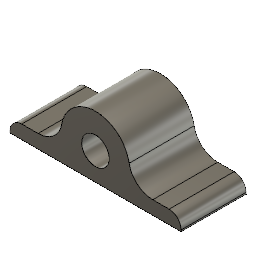
Rod Attach (Autodesk Fusion 360 design; units mm, degrees)
Autodesk Fusion 360 part; units mm, degrees
sketch "Sketch1" plane through (0, 0, 0) normal (0, 0, 1) x (1, 0, 0)
  circle A0 centre (0, 0) radius 4
  circle A1 centre (0, 0) radius 10
  line L0 (-25, -8) -> (25, -8)
  line L1 (25, -8) -> (25, -4)
  line L2 (25, -4) -> (-25, -4)
  line L3 (-25, -4) -> (-25, -8)
  line L4 (-25, -8) -> (25, -4) construction
  line L5 (25, -8) -> (-25, -4) construction
  circle A2 centre (-16.7332, 3) radius 7
  circle A3 centre (16.7332, 3) radius 7
  dimension "d1" = 8
  dimension "d2" = 20
  dimension "d3" = 50
  dimension "d4" = 4
  dimension "d5" = 14
  dimension "d6" = 14
  constraint coincident A0.centre A1.centre
  constraint perpendicular L0 L1
  constraint parallel L0 L2
  constraint parallel L1 L3
  constraint horizontal L0
  constraint tangent L2 A2
  constraint tangent A1 A2
  constraint tangent A1 A3
  constraint tangent L2 A3
  measures "d1" diameter of A0
  measures "d2" diameter of A1
  measures "d3" distance of L1.end L2.end
  measures "d4" distance of L0.end L1.end
  measures "d5" diameter of A2
  measures "d6" diameter of A3
extrude "Extrude1" add sketch "Sketch1" along normal blind 19 contours A1 L2 | A1 L0 L2 | A1 L0 L1 L2 | A1 L2 A3 | A1 L2 A2 | A1 L0 L2 L3
fillet "Fillet1" radius 3.5 2 edges at (25, -4, 9.5) (-25, -4, 9.5)
